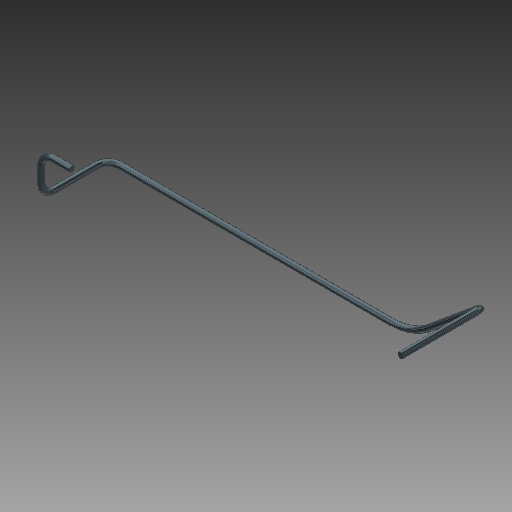
# Autodesk Inventor part: 314-15
Saved by Autodesk Inventor 2019 (Build 230136000, 136)
## iProperties
Company: Autodesk Inc.
Created: 2007-12-31
Part Number: 314-15
Document SubType Name: Modeling
Designer: Autodesk Inc.
Density: 7.85 g/cm^3
Material: Steel
Description: SIDE MOUNTING BAR
Mass: 75.8289 g
Surface Area: 77.6706 cm^2
Volume: 9.65974 cm^3
Appearance: Lead
Component Category: Lower Component
Author: Inventor
Autodesk Inventor part; units mm, degrees
ref_plane "Work Plane1" through (0, 0, -70) normal (0, 0, 1) x (1, 0, 0)
ref_plane "Work Plane2" through (0, -50, 0) normal (0, 1, 0) x (-1, 0, 0)
ref_plane "Work Plane3" through (-310, 0, 0) normal (1, 0, 0) x (0, 1, 0)
sketch "Sketch2" plane through (0, 0, -70) normal (0, 0, 1) x (1, 0, 0)
  line L0 (0, 0) -> (-60, -50) construction
  line L1 (-60, -50) -> (-310, -50) construction
  line L2 (-310, 10) -> (-310, -60) construction
  dimension "d3" = 250
  dimension "d4" = 50
  constraints: 4 end point, 3 coincident, 1 horizontal, 1 point on line
  measures "d3" distance of L0.end L1.end
  measures "d4" distance from line of point (0, 0) L1
sketch "Sketch3" plane through (-310, 0, 0) normal (1, 0, 0) x (0, 1, 0)
  line L0 (-50, -70) -> (-50, -15) construction
  line L1 (-50, -15) -> (-17.5, -15) construction
  dimension "d5" = 55
  dimension "d6" = 32.5
  constraints: 4 end point, 2 coincident, 1 perpendicular, 1 vertical
  measures "d5" distance of L0.start L0.end
  measures "d6" distance of L0.end L1.end
ref_plane "Work Plane4" through (-310, -17.5, -15) normal (0, 1, 0) x (-1, 0, 0)
sketch "Sketch4" plane through (-310, -17.5, -15) normal (0, 1, 0) x (-1, 0, 0)
  line L0 (0, 0) -> (-25, 0) construction
  dimension "d7" = 25
  constraints: 2 end point, 1 coincident, 1 horizontal
  measures "d7" distance of L0.start L0.end
sketch "Sketch5" plane through (0, 0, 0) normal (0, 0, 1) x (1, 0, 0)
  circle A0 centre (0, 0) radius 2.5
  dimension "d13" = 5
  constraints: 1 centre point, 1 coincident
  measures "d13" diameter of A0
sketch3d "3D Sketch1"
  line L0 (0, 0, 0) -> (0, 0, -60)
  arc A0 (0, 0, -60) -> (-7.6822, -6.4018, -70) centre (-7.6822, -6.4018, -60) ccw
  line L1 (-7.6822, -6.4018, -70) -> (-46.0933, -38.4111, -70)
  arc A1 (-46.0933, -38.4111, -70) -> (-78.1025, -50, -70) centre (-78.1025, 0, -70) ccw
  line L2 (-78.1025, -50, -70) -> (-300, -50, -70)
  arc A2 (-300, -50, -70) -> (-310, -50, -60) centre (-300, -50, -60) ccw
  line L3 (-310, -50, -60) -> (-310, -50, -25)
  arc A3 (-310, -50, -25) -> (-310, -40, -15) centre (-310, -40, -25) ccw
  line L4 (-310, -40, -15) -> (-310, -27.5, -15)
  arc A4 (-310, -27.5, -15) -> (-300, -17.5, -15) centre (-300, -27.5, -15) ccw
  line L5 (-300, -17.5, -15) -> (-285, -17.5, -15)
  dimension "d8" = 10
  dimension "d9" = 10
  dimension "d10" = 10
  dimension "d11" = 10
  dimension "d12" = 50
sweep "Sweep1" add profiles "Sketch5" path "3D Sketch1"
equation "\"d9\" = d8"
equation "\"d10\" = d8"
equation "\"d11\" = d8"
body "Solid1"
